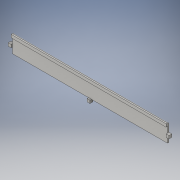
# Autodesk Inventor part: Arm Side
Saved by Autodesk Inventor 2016 (Build 200138000, 138)
## iProperties
Created: 2016-04-25
Part Number: Arm Side
Material: PVC-Piping
Document SubType Name: Modeling
Designer: rubenjm
Density: 1.4 g/cm^3
Appearance: Smooth - White
Author: rubenjm
Autodesk Inventor part; units mm, degrees
ref_plane "YZ Plane" through (0, 0, 0) normal (1, 0, 0) x (0, 1, 0)
ref_plane "XZ Plane" through (0, 0, 0) normal (0, 1, 0) x (-1, 0, 0)
ref_plane "XY Plane" through (0, 0, 0) normal (0, 0, 1) x (1, 0, 0)
sketch "Sketch1" plane through (0, 0, 0) normal (0, 0, 1) x (1, 0, 0)
  line L0 (673.1, 76.2) -> (0, 76.2)
  line L1 (0, 25.4) -> (-12.7, 25.4)
  line L2 (-12.7, 25.4) -> (-12.7, 38.1)
  line L3 (-12.7, 38.1) -> (0, 38.1)
  line L4 (0, 76.2) -> (0, 38.1)
  line L5 (0, 25.4) -> (0, 0)
  line L6 (336.55, 12.7) -> (336.55, 76.2) construction
  line L7 (673.1, 25.4) -> (685.8, 25.4)
  line L8 (685.8, 25.4) -> (685.8, 38.1)
  line L9 (685.8, 38.1) -> (673.1, 38.1)
  line L10 (673.1, 0) -> (673.1, 25.4)
  line L11 (673.1, 38.1) -> (673.1, 76.2)
  line L12 (342.9, -12.7) -> (330.2, -12.7)
  line L13 (330.2, -12.7) -> (330.2, 0)
  line L14 (342.9, 0) -> (342.9, -12.7)
  line L15 (330.2, 0) -> (342.9, 0) construction
  line L16 (336.55, 0) -> (336.55, -12.7) construction
  line L17 (0, 0) -> (330.2, 0)
  line L18 (342.9, 0) -> (673.1, 0)
  point P0 (0, 34.925)
  point P1 (673.1, 34.925)
  dimension "d0" = 673.1
  dimension "d1" = 76.2
  dimension "d9" = 12.7
  dimension "d12" = 12.7
  dimension "d16" = 12.7
  dimension "d17" = 25.4
  dimension "d19" = 25.4
  constraints: 38 end point, 6 parallel, 5 symmetric about line, 4 horizontal, 3 midpoint, 3 perpendicular, 1 collinear
  measures "d0" distance of L0.end L0.start
  measures "d1" distance of L0.start L10.start
  measures "d9" distance of L1.end L2.end
  measures "d12" distance of L14.start L12.start
  measures "d16" distance of L2.end L3.end
  measures "d17" distance of L1.start L5.end
  measures "d19" distance of L10.start L7.start
extrude "Extrusion1" add sketch "Sketch1" along normal blind 12.7
sketch "Sketch2" plane through (0, 0, 12.7) normal (0, 0, 1) x (1, 0, 0)
  line L0 (0, 0) -> (673.1, 0)
  line L1 (673.1, 0) -> (673.1, 63.5)
  line L2 (673.1, 63.5) -> (0, 63.5)
  line L3 (0, 63.5) -> (0, 0)
  dimension "d4" = 673.1
  dimension "d5" = 63.5
  constraints: 8 end point, 2 parallel, 1 horizontal, 1 perpendicular
  measures "d4" distance of L2.end L1.end
  measures "d5" distance of L1.end L0.end
extrude "Extrusion2" cut sketch "Sketch2" against normal blind 6.35
fillet "Fillet1" radius 6.35 1 edges at (336.55, 76.2, 0)
equation "\"d19\" = d17"
body "Solid1"
